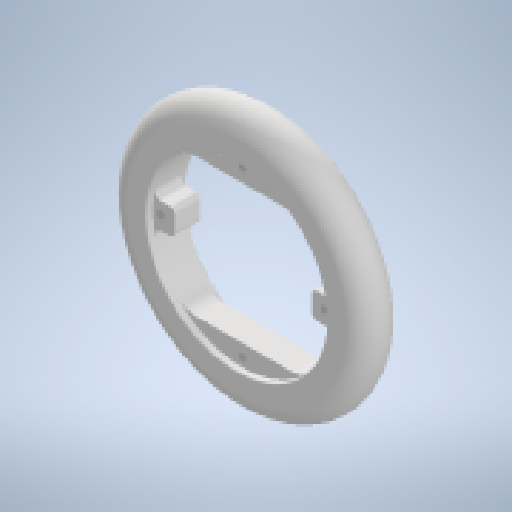
# Autodesk Inventor part: steering wheel
Saved by Autodesk Inventor 2025 (Build 290162000, 162)
## iProperties
Created: 2025-01-07
Part Number: steering wheel
Material: Generic
Document SubType Name: Modeling
Designer: 5014070
Density: 1 g/cm^3
Appearance: Default
Author: 5014070
Autodesk Inventor part; units mm, degrees
ref_plane "YZ Plane" through (0, 0, 0) normal (1, 0, 0) x (0, 1, 0)
ref_plane "XZ Plane" through (0, 0, 0) normal (0, 1, 0) x (-1, 0, 0)
ref_plane "XY Plane" through (0, 0, 0) normal (0, 0, 1) x (1, 0, 0)
sketch "Sketch2" plane through (0, 0, 0) normal (0, 0, 1) x (1, 0, 0)
  circle A0 centre (0, 0) radius 100
  arc A1 (-69.282, 10) -> (-69.282, -10) centre (0, 0) ccw
  line L0 (-63.2456, -10) -> (-45, -10)
  line L1 (70, 10) -> (69.282, 10)
  line L2 (-70, -10) -> (-69.2965, -9.8995) construction
  line L3 (70, -10) -> (-69.2965, 9.8995) construction
  line L4 (-40, -70) -> (40, 70) construction
  line L5 (-40, 70) -> (40, -70) construction
  arc A2 (-48.4615, 50.5122) -> (-68.1106, 16.1538) centre (0, 0) ccw
  arc A3 (-40, -57.4456) -> (40, -57.4456) centre (0, 0) ccw
  arc A4 (-68.1106, -16.1538) -> (-48.4615, -50.5122) centre (0, 0) ccw
  line L6 (-40, -46.9042) -> (-40, -15)
  arc A5 (48.4615, -50.5122) -> (68.1106, -16.1538) centre (0, 0) ccw
  line L7 (40, 46.9042) -> (40, 15)
  arc A6 (40, 57.4456) -> (-40, 57.4456) centre (0, 0) ccw
  arc A7 (-40, 46.9042) -> (-48.4615, 50.5122) centre (-45, 46.9042) ccw
  line L8 (-40, 15) -> (-40, 46.9042)
  line L9 (-45, 10) -> (-63.2456, 10)
  line L10 (-69.2965, 9.8995) -> (-70, 10) construction
  arc A8 (68.1106, 16.1538) -> (48.4615, 50.5122) centre (0, 0) ccw
  arc A9 (69.282, -10) -> (69.282, 10) centre (0, 0) ccw
  line L11 (69.282, -10) -> (70, -10)
  line L12 (63.2456, 10) -> (45, 10)
  line L13 (45, -10) -> (63.2456, -10)
  line L14 (40, -15) -> (40, -46.9042)
  line L15 (-69.282, 10) -> (-70, 10)
  line L16 (-69.2965, -9.8995) -> (70, 10) construction
  arc A10 (-68.1106, 16.1538) -> (-63.2456, 10) centre (-63.2456, 15) ccw
  arc A11 (-45, 10) -> (-40, 15) centre (-45, 15) ccw
  arc A12 (-48.4615, -50.5122) -> (-40, -46.9042) centre (-45, -46.9042) ccw
  arc A13 (-40, -15) -> (-45, -10) centre (-45, -15) ccw
  arc A14 (-63.2456, -10) -> (-68.1106, -16.1538) centre (-63.2456, -15) ccw
  arc A15 (40, -46.9042) -> (48.4615, -50.5122) centre (45, -46.9042) ccw
  arc A16 (68.1106, -16.1538) -> (63.2456, -10) centre (63.2456, -15) ccw
  arc A17 (45, -10) -> (40, -15) centre (45, -15) ccw
  arc A18 (40, 15) -> (45, 10) centre (45, 15) ccw
  arc A19 (63.2456, 10) -> (68.1106, 16.1538) centre (63.2456, 15) ccw
  arc A20 (48.4615, 50.5122) -> (40, 46.9042) centre (45, 46.9042) ccw
  line L17 (-40, -57.4456) -> (40, -57.4456)
  line L18 (40, 57.4456) -> (-40, 57.4456)
  line L19 (53.2456, 10) -> (53.2456, -10)
  line L20 (-53.2456, 10) -> (-53.2456, -10)
  circle A21 centre (0, 0) radius 70
  circle A22 centre (-63.2456, 0) radius 3
  circle A23 centre (63.2456, 0) radius 3
  line L21 (0, -57.4456) -> (0, -70)
  circle A24 centre (0, -63.7228) radius 3
  line L22 (0, 70) -> (0, 57.4456)
  circle A25 centre (0, 63.7228) radius 3
  line L23 (-63.2456, 0) -> (-53.2456, 0)
  line L24 (-63.2456, 0) -> (0, 0)
  line L25 (63.2456, 0) -> (53.2456, 0)
  line L26 (63.2456, 0) -> (0, 0)
  line L27 (0, 63.7228) -> (0, 53.7228)
  line L28 (0, 53.7228) -> (-44.876, 53.7228)
  line L29 (0, 53.7228) -> (44.876, 53.7228)
  line L30 (0, -63.7228) -> (0, -53.7228)
  line L31 (0, -53.7228) -> (44.876, -53.7228)
  line L32 (0, -53.7228) -> (-44.876, -53.7228)
  point P0 (68.1106, -16.1538)
  point P1 (69.282, -10)
  point P2 (68.1106, 16.1538)
  point P3 (48.4615, 50.5122)
  point P4 (-40, 57.4456)
  point P5 (-68.1106, 16.1538)
  point P6 (-69.282, 10)
  point P7 (-69.282, -10)
  point P8 (-48.4615, -50.5122)
  point P9 (-40, 57.4456)
  point P10 (53.2456, -10)
  point P11 (-68.1106, 16.1538)
  point P12 (48.4615, 50.5122)
  point P13 (68.1106, 16.1538)
  point P14 (68.1106, -16.1538)
  point P15 (-48.4615, -50.5122)
  dimension "d0" = 200
  dimension "d1" = 140
  dimension "d2" = 20
  dimension "d3" = 80
  dimension "d4" = 5
  dimension "d5" = 5
  dimension "d6" = 5
  dimension "d13" = 6
  dimension "d14" = 6
  dimension "d15" = 6
  dimension "d18" = 6
  dimension "d34" = 10
  dimension "d35" = 10
  dimension "d36" = 63.2455
  dimension "d37" = 18.2456
  dimension "d38" = 18.2456
  dimension "d43" = 10
  dimension "d44" = 10
  constraints: 66 end point, 52 point on circle, 25 centre point, 25 tangent, 17 parallel, 16 point on line, 9 equal radius, 9 midpoint, 8 horizontal, 2 coincident, 2 perpendicular, 1 collinear, 1 vertical, 8 other
  measures "d0" diameter of A0
  measures "d1" diameter of A1
  measures "d2" distance of L1.start L3.start
  measures "d3" distance of L5.start L4.end
  measures "d4" radius of A7
  measures "d5" radius of A10
  measures "d6" radius of A11
  measures "d13" diameter of A22
  measures "d14" diameter of A23
  measures "d15" diameter of A24
  measures "d18" diameter of A25
  measures "d34" distance of L23.start L23.end
  measures "d35" distance of L25.start L25.end
  measures "d36" distance of L25.start L24.end
  measures "d37" distance of L13.start L13.end
  measures "d38" distance of L0.start L0.end
  measures "d43" distance of L27.start L27.end
  measures "d44" distance of L30.start L30.end
extrude "Extrusion1" add sketch "Sketch2" along normal blind 30 contours A0
extrude "Extrusion5" add sketch "Sketch2" along normal blind 25 contours A21 A10 L9 L20 L0 A14 A1 | A21 L18 L27 L28 | L32 L30 L17 A21 | A6 L22 A25 L18 | L27 L18 A21 L29 | L17 L21 A24 A3 | L31 A21 L17 L30 | A6 L18 L22 A25 | L21 A24 L17 A3 | L19 L12 A19 A21 A9 A16 L13 | A24 L21 | L21 A24
extrude "Extrusion2" cut sketch "Sketch2" along normal blind 5 contours A21 A10 L9 L20 L0 A14 A1 | A21 L28 L29 A20 L7 A18 L12 L19 L26 L24 L20 L9 A11 L8 A7 | A12 L6 A13 L0 L20 L24 L26 L19 L13 A17 L14 A15 A21 L31 L32 | A21 L18 L27 L28 | L32 L30 L17 A21 | A6 L22 A25 L18 | L27 L18 A21 L29 | L17 L21 A24 A3 | L31 A21 L17 L30 | A6 L18 L22 A25 | L21 A24 L17 A3 | A25 L22 | L22 A25 | L19 L12 A19 A21 A9 A16 L13 | A24 L21 | L21 A24 | A22 | A23
extrude "Extrusion3" cut sketch "Sketch2" along normal through all contours A21 L28 L29 A20 L7 A18 L12 L19 L26 L24 L20 L9 A11 L8 A7 | A12 L6 A13 L0 L20 L24 L26 L19 L13 A17 L14 A15 A21 L31 L32 | A24 L21 | L21 A24
extrude "Extrusion4" cut sketch "Sketch2" along normal blind 200 contours A25 L22 | L22 A25 | A24 L21 | L21 A24 | A22 | A23
thread "Thread2" size "M6x1" class "6H" standard "ANSI Metric M Profile" full length
thread "Thread4" size "M6x1" class "6H" standard "ANSI Metric M Profile" full length
fillet "Fillet4" radius 1 29 edges at (-60.765, -34.7507, 0) (-46.6964, -52.1483, 0) (-42.4788, -55.6377, 0) (0, -70, 0) (42.4788, -55.6377, 0) (46.6964, -52.1483, 0) (60.765, -34.7507, 0) (68.7652, -13.09, 0) (70, 0, 0) (68.7652, 13.09, 0) (60.765, 34.7507, 0) (46.6964, 52.1483, 0) (42.4788, 55.6377, 0) (0, 70, 0) (-42.4788, 55.6377, 0) (-46.6964, 52.1483, 0) (-60.765, 34.7507, 0) (-68.7652, 13.09, 0) (-70, 0, 0) (-68.7652, -13.09, 0) (67.1443, -19.79, 30) (46.6964, -52.1483, 30) (0, -70, 30) (-46.6964, -52.1483, 30) (-70, 0, 30) (-46.6964, 52.1483, 30) (0, 70, 30) (46.6964, 52.1483, 30) (60.765, 34.7507, 30)
fillet "Fillet5" radius 15 2 edges at (-100, 0, 0) (-100, 0, 30)
fillet "Fillet6" radius 4 4 edges at (53.2456, -10, 15) (53.2456, 10, 15) (-53.2456, 10, 15) (-53.2456, -10, 15)
sketch "Sketch3" plane through (0, 0, 30) normal (0, 0, 1) x (1, 0, 0)
  circle A0 centre (-63.2456, 0) radius 3 projected
  circle A1 centre (0, 63.7228) radius 2.9 projected
  line L0 (-63.2456, 0) -> (0, 63.7228)
  circle A2 centre (63.2456, 0) radius 3 projected
  line L1 (0, 63.7228) -> (63.2456, 0)
  line L2 (63.2456, 0) -> (0, -63.7228)
  line L3 (0, -63.7228) -> (-63.2456, 0)
  point P0 (0, 0)
  constraints: 8 end point, 2 parallel
thread "Thread6" size "M6x1" class "6H" standard "ANSI Metric M Profile" full length
thread "Thread7" size "M6x1" class "6H" standard "ANSI Metric M Profile" full length
fillet "Fillet9" radius 20 4 edges at (44.876, -53.7228, 15) (-44.876, -53.7228, 15) (-44.876, 53.7228, 15) (44.876, 53.7228, 15)
equation "\"d16\" = d0"
body "Solid1"
